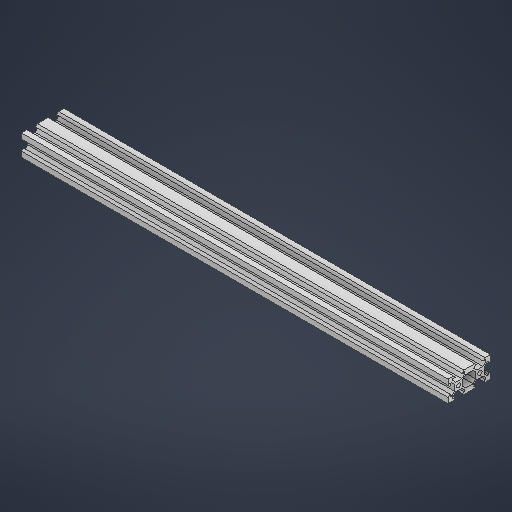
# Autodesk Inventor part: V Extrustion 40x400mm
Saved by Autodesk Inventor 2025.1 (Build 291241000, 241)
## iProperties
Created: 2024-11-10
Part Number: V Extrustion 40x400mm
Material: Generic
Document SubType Name: Modeling
Designer: jerem
Density: 1 g/cm^3
Appearance: Default
Author: jerem
Autodesk Inventor part; units mm, degrees
ref_plane "YZ Plane" through (0, 0, 0) normal (1, 0, 0) x (0, 1, 0)
ref_plane "XZ Plane" through (0, 0, 0) normal (0, 1, 0) x (-1, 0, 0)
ref_plane "XY Plane" through (0, 0, 0) normal (0, 0, 1) x (1, 0, 0)
sketch "Sketch1" plane through (0, 0, 0) normal (1, 0, 0) x (0, 1, 0)
  line L0 (-9.95, 0) -> (9.95, 0) construction
  line L1 (9.95, 19.9) -> (-9.95, 19.9) construction
  line L2 (-9.95, 19.9) -> (-9.95, 0) construction
  line L3 (-9.95, 0) -> (9.95, 19.9) construction
  line L4 (9.95, 0) -> (-9.95, 19.9) construction
  line L5 (9.95, 14.875) -> (8.15, 13.075)
  line L6 (8.15, 13.075) -> (8.15, 15.3893)
  line L7 (8.15, 15.3893) -> (6.5, 15.3893)
  line L8 (6.5, 15.3893) -> (3.9107, 12.8)
  line L9 (3.9107, 12.8) -> (3.9107, 9.95)
  line L10 (9.95, 5.025) -> (8.15, 6.825)
  line L11 (8.15, 6.825) -> (8.15, 4.5107)
  line L12 (3.9107, 7.1) -> (3.9107, 9.95)
  line L13 (0, 9.95) -> (10.8561, 9.95) construction
  line L14 (8.15, 4.5107) -> (6.5, 4.5107)
  line L15 (6.5, 4.5107) -> (3.9107, 7.1)
  circle A0 centre (0, 9.95) radius 2
  line L16 (9.95, 0) -> (9.95, 5.025)
  line L17 (9.95, 14.875) -> (9.95, 19.9)
  line L18 (-4.925, 19.9) -> (-9.95, 19.9)
  line L19 (-4.925, 19.9) -> (-3.125, 18.1)
  line L20 (-5.4393, 16.45) -> (-2.85, 13.8607)
  line L21 (-5.4393, 18.1) -> (-5.4393, 16.45)
  line L22 (-3.125, 18.1) -> (-5.4393, 18.1)
  line L23 (-2.85, 13.8607) -> (0, 13.8607)
  line L24 (2.85, 13.8607) -> (0, 13.8607)
  line L25 (5.4393, 16.45) -> (2.85, 13.8607)
  line L26 (5.4393, 18.1) -> (5.4393, 16.45)
  line L27 (3.125, 18.1) -> (5.4393, 18.1)
  line L28 (4.925, 19.9) -> (3.125, 18.1)
  line L29 (9.95, 19.9) -> (4.925, 19.9)
  line L30 (-9.95, 5.025) -> (-9.95, 0)
  line L31 (-9.95, 5.025) -> (-8.15, 6.825)
  line L32 (-6.5, 4.5107) -> (-3.9107, 7.1)
  line L33 (-8.15, 4.5107) -> (-6.5, 4.5107)
  line L34 (-8.15, 6.825) -> (-8.15, 4.5107)
  line L35 (-3.9107, 7.1) -> (-3.9107, 9.95)
  line L36 (-3.9107, 12.8) -> (-3.9107, 9.95)
  line L37 (-6.5, 15.3893) -> (-3.9107, 12.8)
  line L38 (-8.15, 15.3893) -> (-6.5, 15.3893)
  line L39 (-8.15, 13.075) -> (-8.15, 15.3893)
  line L40 (-9.95, 14.875) -> (-8.15, 13.075)
  line L41 (-9.95, 19.9) -> (-9.95, 14.875)
  line L42 (4.925, 0) -> (9.95, 0)
  line L43 (4.925, 0) -> (3.125, 1.8)
  line L44 (5.4393, 3.45) -> (2.85, 6.0393)
  line L45 (5.4393, 1.8) -> (5.4393, 3.45)
  line L46 (3.125, 1.8) -> (5.4393, 1.8)
  line L47 (2.85, 6.0393) -> (0, 6.0393)
  line L48 (-2.85, 6.0393) -> (0, 6.0393)
  line L49 (-5.4393, 3.45) -> (-2.85, 6.0393)
  line L50 (-5.4393, 1.8) -> (-5.4393, 3.45)
  line L51 (-3.125, 1.8) -> (-5.4393, 1.8)
  line L52 (-4.925, 0) -> (-3.125, 1.8)
  line L53 (-9.95, 0) -> (-4.925, 0)
  line L54 (-9.95, -19.9) -> (9.95, -19.9) construction
  line L55 (9.95, 0) -> (-9.95, 0) construction
  line L56 (-9.95, 0) -> (-9.95, -19.9) construction
  line L57 (-9.95, -19.9) -> (9.95, 0) construction
  line L58 (9.95, -19.9) -> (-9.95, 0) construction
  line L59 (9.95, -5.025) -> (8.15, -6.825)
  line L60 (8.15, -6.825) -> (8.15, -4.5107)
  line L61 (8.15, -4.5107) -> (6.5, -4.5107)
  line L62 (6.5, -4.5107) -> (3.9107, -7.1)
  line L63 (3.9107, -7.1) -> (3.9107, -9.95)
  line L64 (9.95, -14.875) -> (8.15, -13.075)
  line L65 (8.15, -13.075) -> (8.15, -15.3893)
  line L66 (3.9107, -12.8) -> (3.9107, -9.95)
  line L67 (0, -9.95) -> (11.144, -9.95) construction
  line L68 (8.15, -15.3893) -> (6.5, -15.3893)
  line L69 (6.5, -15.3893) -> (3.9107, -12.8)
  circle A1 centre (0, -9.95) radius 2
  line L70 (9.95, -19.9) -> (9.95, -14.875)
  line L71 (9.95, -5.025) -> (9.95, 0)
  line L72 (-4.925, 0) -> (-9.95, 0)
  line L73 (-4.925, 0) -> (-3.125, -1.8)
  line L74 (-5.4393, -3.45) -> (-2.85, -6.0393)
  line L75 (-5.4393, -1.8) -> (-5.4393, -3.45)
  line L76 (-3.125, -1.8) -> (-5.4393, -1.8)
  line L77 (-2.85, -6.0393) -> (0, -6.0393)
  line L78 (2.85, -6.0393) -> (0, -6.0393)
  line L79 (5.4393, -3.45) -> (2.85, -6.0393)
  line L80 (5.4393, -1.8) -> (5.4393, -3.45)
  line L81 (3.125, -1.8) -> (5.4393, -1.8)
  line L82 (4.925, 0) -> (3.125, -1.8)
  line L83 (9.95, 0) -> (4.925, 0)
  line L84 (-9.95, -14.875) -> (-9.95, -19.9)
  line L85 (-9.95, -14.875) -> (-8.15, -13.075)
  line L86 (-6.5, -15.3893) -> (-3.9107, -12.8)
  line L87 (-8.15, -15.3893) -> (-6.5, -15.3893)
  line L88 (-8.15, -13.075) -> (-8.15, -15.3893)
  line L89 (-3.9107, -12.8) -> (-3.9107, -9.95)
  line L90 (-3.9107, -7.1) -> (-3.9107, -9.95)
  line L91 (-6.5, -4.5107) -> (-3.9107, -7.1)
  line L92 (-8.15, -4.5107) -> (-6.5, -4.5107)
  line L93 (-8.15, -6.825) -> (-8.15, -4.5107)
  line L94 (-9.95, -5.025) -> (-8.15, -6.825)
  line L95 (-9.95, 0) -> (-9.95, -5.025)
  line L96 (4.925, -19.9) -> (9.95, -19.9)
  line L97 (4.925, -19.9) -> (3.125, -18.1)
  line L98 (5.4393, -16.45) -> (2.85, -13.8607)
  line L99 (5.4393, -18.1) -> (5.4393, -16.45)
  line L100 (3.125, -18.1) -> (5.4393, -18.1)
  line L101 (2.85, -13.8607) -> (0, -13.8607)
  line L102 (-2.85, -13.8607) -> (0, -13.8607)
  line L103 (-5.4393, -16.45) -> (-2.85, -13.8607)
  line L104 (-5.4393, -18.1) -> (-5.4393, -16.45)
  line L105 (-3.125, -18.1) -> (-5.4393, -18.1)
  line L106 (-4.925, -19.9) -> (-3.125, -18.1)
  line L107 (-9.95, -19.9) -> (-4.925, -19.9)
  line L108 (5.4393, -1.8) -> (5.4393, 1.8)
  line L109 (-5.4393, 1.8) -> (-5.4393, -1.8)
  point P0 (0, 0)
  point P1 (0, 0)
  dimension "d2" = 19.9
  dimension "d3" = 19.9
  dimension "d4" = 6.25
  dimension "d5" = 5.7
  dimension "d6" = 0.75
  dimension "d7" = 4
  dimension "d8" = 1.8
  dimension "d9" = 45
  dimension "d10" = 1.65
  dimension "d11" = 360
  dimension "d14" = 19.9
  dimension "d15" = 19.9
  dimension "d16" = 6.25
  dimension "d17" = 5.7
  dimension "d18" = 0.75
  dimension "d19" = 4
  dimension "d20" = 1.8
  dimension "d21" = 45
  dimension "d22" = 1.65
  dimension "d23" = 360
  constraints: 220 end point, 12 parallel, 10 equal length, 6 horizontal, 6 perpendicular, 6 vertical, 5 midpoint, 4 coincident, 2 centre point, 2 point on line, 202 other
  measures "d2" distance of L2.start L1.start
  measures "d3" distance of L1.start L0.end
  measures "d4" distance of L11.start L5.end
  measures "d5" distance of L12.start L9.start
  measures "d6" distance between parallel lines of L3 L8
  measures "d7" diameter of A0
  measures "d8" distance between parallel lines of L6 L17
  measures "d9" angle of L6 L5
  measures "d10" distance from line of L7.end L6
  measures "d14" distance of L56.start L55.start
  measures "d15" distance of L55.start L54.end
  measures "d16" distance of L65.start L59.end
  measures "d17" distance of L66.start L63.start
  measures "d18" distance between parallel lines of L57 L62
  measures "d19" diameter of A1
  measures "d20" distance between parallel lines of L60 L71
  measures "d21" angle of L60 L59
  measures "d22" distance from line of L61.end L60
extrude "Extrusion1" add sketch "Sketch1" along normal blind 400 contours L5 L6 L7 L8 L9 L12 L15 L14 L11 L10 L16 L42 L108 L45 L44 L47 L48 L49 L50 L109 L53 L30 L31 L34 L33 L32 L35 L36 L37 L38 L39 L40 L41 L18 L19 L22 L21 L20 L23 L24 L25 L26 L27 L28 L29 L17 | L71 L59 L60 L61 L62 L63 L66 L69 L68 L65 L64 L70 L96 L97 L100 L99 L98 L101 L102 L103 L104 L105 L106 L107 L84 L85 L88 L87 L86 L89 L90 L91 L92 L93 L94 L95 L53 L109 L75 L74 L77 L78 L79 L80 L108 L42
equation "\"d3\" = d15"
body "Solid1"
